Autodesk Fusion 360 part; units mm, degrees
(part 2 of 2)
sketch "Sketch53" plane through (0, 12.5, 0) normal (0, 1, 0) x (-1, 0, 0)
  circle A0 centre (-41, 14.5) radius 4.5
  line L0 (-2.4975, 53.5) -> (-2.4975, 22.5658)
  arc A1 (-31.7708, 34.6912) -> (-2.4975, 22.5658) centre (0.0025, 70) ccw
  line L1 (-31.7708, 34.6912) -> (-12.962, 53.5)
  line L2 (-12.962, 53.5) -> (-2.4975, 53.5)
  line L3 (12.9669, 53.5) -> (31.7757, 34.6912)
  arc A2 (2.5025, 22.5658) -> (31.7757, 34.6912) centre (0.0025, 70) ccw
  line L4 (2.5025, 22.5658) -> (2.5025, 53.5)
  line L5 (2.5025, 53.5) -> (12.9669, 53.5)
  line L6 (16.5025, 82.9645) -> (35.3113, 101.7733)
  arc A3 (47.4366, 72.5) -> (35.3113, 101.7733) centre (0.0025, 70) ccw
  line L7 (47.4366, 72.5) -> (16.5025, 72.5)
  line L8 (16.5025, 72.5) -> (16.5025, 82.9645)
  line L9 (-2.4975, 117.4342) -> (-2.4975, 86.5)
  line L10 (-2.4975, 86.5) -> (-12.962, 86.5)
  line L11 (-12.962, 86.5) -> (-31.7708, 105.3088)
  arc A4 (-2.4975, 117.4342) -> (-31.7708, 105.3088) centre (0.0025, 70) ccw
  line L12 (2.5025, 86.5) -> (2.5025, 117.4342)
  arc A5 (31.7757, 105.3088) -> (2.5025, 117.4342) centre (0.0025, 70) ccw
  line L13 (31.7757, 105.3088) -> (12.9669, 86.5)
  line L14 (12.9669, 86.5) -> (2.5025, 86.5)
  arc A6 (35.3113, 38.2267) -> (47.4366, 67.5) centre (0.0025, 70) ccw
  line L15 (35.3113, 38.2267) -> (16.5025, 57.0355)
  line L16 (16.5025, 57.0355) -> (16.5025, 67.5)
  line L17 (16.5025, 67.5) -> (47.4366, 67.5)
  line L18 (-47.4317, 67.5) -> (-16.4975, 67.5)
  line L19 (-16.4975, 67.5) -> (-16.4975, 57.0355)
  line L20 (-16.4975, 57.0355) -> (-35.3063, 38.2267)
  arc A7 (-47.4317, 67.5) -> (-35.3063, 38.2267) centre (0.0025, 70) ccw
  arc A8 (-35.3063, 101.7733) -> (-47.4317, 72.5) centre (0.0025, 70) ccw
  line L21 (-35.3063, 101.7733) -> (-16.4975, 82.9645)
  line L22 (-16.4975, 82.9645) -> (-16.4975, 72.5)
  line L23 (-16.4975, 72.5) -> (-47.4317, 72.5)
  line L24 (-50, 90) -> (-50, 0)
  line L25 (-50, 0) -> (53, 0)
  line L26 (53, 0) -> (53, 90)
  line L27 (53, 90) -> (50, 90)
  arc A9 (50, 90) -> (20, 120) centre (20, 90) ccw
  line L28 (20, 120) -> (-20, 120)
  arc A10 (-20, 120) -> (-50, 90) centre (-20, 90) ccw
  line L29 (50, 90) -> (58, 90)
  line L30 (58, 90) -> (58, 0)
  line L31 (58, 0) -> (50, 0)
  line L32 (50, 0) -> (50, 90)
  constraint horizontal L29
  constraint vertical L30
  constraint horizontal L31
  constraint vertical L32
  constraint coincident L27.end A9.start
extrude "Extrude57" add sketch "Sketch53" along normal blind 3 contours L25 L26 L27 L29 L31 L32 | L26 L29 L30 L31 bodies 1
sketch "Sketch54" plane through (0, 12.5, 0) normal (0, -1, 0) x (1, 0, 0)
  line L0 (-53, 0) -> (-53, 90)
  line L1 (-53, 90) -> (-58, 90)
  line L2 (-58, 90) -> (-58, 0)
  line L3 (-58, 0) -> (-53, 0)
  line L4 (-57.5, 90) -> (-55.5, 90)
  line L5 (-55.5, 90) -> (-55.5, 0)
  line L6 (-55.5, 0) -> (-57.5, 0)
  line L7 (-57.5, 0) -> (-57.5, 90)
  dimension "d272" = 0.5
  constraint perpendicular L4 L5
  constraint parallel L4 L6
  constraint parallel L5 L7
  constraint coincident L1 L4.end
  constraint coincident L1 L4.start
  measures "d272" distance of L2 L7
extrude "Extrude58" cut 1 faces at (53.8333, 12.5, 30) along direction (0, 1, 0) blind 1 on bodies 1 bodies 1
extrude "Extrude59" cut 1 faces at (57.6667, 12.5, 60) along direction (0, 1, 0) blind 1 on bodies 1 bodies 1
extrude "Extrude60" cut 1 faces at (54.6667, -12.5, 30) along direction (0, -1, 0) blind 1 on bodies 1 bodies 1
extrude "Extrude61" cut 1 faces at (57.6667, -12.5, 30) along direction (0, -1, 0) blind 1 on bodies 1 bodies 1
sketch "Sketch55" plane through (-50, 0, 0) normal (-1, 0, 0) x (0, -1, 0)
  line L0 (-10.5, 90) -> (-10.5, 0)
  line L1 (-10.5, 0) -> (10.5, 0)
  line L2 (10.5, 0) -> (10.5, 90)
  line L3 (10.5, 90) -> (-10.5, 90)
  line L4 (7.5, 30) -> (-7.5, 30)
  arc A0 (-7.5, 35) -> (-7.5, 30) centre (-7.5, 32.5) ccw
  line L5 (-7.5, 35) -> (7.5, 35)
  arc A1 (7.5, 30) -> (7.5, 35) centre (7.5, 32.5) ccw
  line L6 (-10.5, 2) -> (10.5, 2)
  dimension "d281" = 2
  constraint coincident L0 L6.start
  constraint coincident L2 L6.end
  constraint perpendicular L2 L6
  measures "d281" distance of L1 L6
extrude "Extrude62" add sketch "Sketch55" along normal blind 2 contours L0 L1 L2 L6 bodies 1
extrude "Extrude63" add 1 faces at (-52, 3.5, 0.6667) along direction (-1, 0, 0) blind 1 on bodies 1 bodies 1
sketch "Sketch56" plane through (76.5769, 0, 0) normal (1, 0, 0) x (0, 1, 0)
  line L0 (-61.7702, 35) -> (-46.7702, 35)
  arc A0 (-46.7702, 30) -> (-46.7702, 35) centre (-46.7702, 32.5) ccw
  line L1 (-46.7702, 30) -> (-61.7702, 30)
  arc A1 (-61.7702, 35) -> (-61.7702, 30) centre (-61.7702, 32.5) ccw
  line L2 (-46.7702, 75) -> (-61.7702, 75)
  arc A2 (-61.7702, 80) -> (-61.7702, 75) centre (-61.7702, 77.5) ccw
  line L3 (-61.7702, 80) -> (-46.7702, 80)
  arc A3 (-46.7702, 75) -> (-46.7702, 80) centre (-46.7702, 77.5) ccw
  line L4 (-61.7702, 50) -> (-46.7702, 50)
  arc A4 (-46.7702, 45) -> (-46.7702, 50) centre (-46.7702, 47.5) ccw
  line L5 (-46.7702, 45) -> (-61.7702, 45)
  arc A5 (-61.7702, 50) -> (-61.7702, 45) centre (-61.7702, 47.5) ccw
  line L6 (-61.7702, 65) -> (-46.7702, 65)
  arc A6 (-46.7702, 60) -> (-46.7702, 65) centre (-46.7702, 62.5) ccw
  line L7 (-46.7702, 60) -> (-61.7702, 60)
  arc A7 (-61.7702, 65) -> (-61.7702, 60) centre (-61.7702, 62.5) ccw
  line L8 (-66.7673, 2) -> (-64.7673, 2)
  line L9 (-64.7673, 2) -> (-64.7673, 25)
  line L10 (-64.7673, 25) -> (-43.7673, 25)
  line L11 (-43.7673, 25) -> (-43.7673, 2)
  line L12 (-43.7673, 2) -> (-41.7673, 2)
  line L13 (-41.7673, 2) -> (-41.7673, 85)
  arc A8 (-41.7673, 85) -> (-46.7673, 90) centre (-46.7673, 85) ccw
  line L14 (-46.7673, 90) -> (-61.7673, 90)
  arc A9 (-61.7673, 90) -> (-66.7673, 85) centre (-61.7673, 85) ccw
  line L15 (-66.7673, 85) -> (-66.7673, 2)
  line L16 (25, 44) -> (39, 44)
  line L17 (39, 40) -> (25, 40)
  arc A10 (39, 40) -> (39, 44) centre (39, 42) ccw
  arc A11 (25, 44) -> (25, 40) centre (25, 42) ccw
  dimension "d286" = 2
  constraint horizontal L16
  constraint horizontal L17
  constraint tangent L16 A10
  constraint tangent L17 A10
  constraint tangent L16 A11
  constraint tangent L17 A11
  measures "d286" radius of A10
extrude "Extrude64" add sketch "Sketch56" along normal blind 16 contours L16 L17 A10 A11 bodies 6 makes body 9
sketch "Sketch57" plane through (0, 0, 44) normal (0, 0, 1) x (-1, 0, 0)
  line L0 (-76.5769, -25) -> (-92.5769, -25)
  line L1 (-92.5769, -25) -> (-92.5769, -39)
  line L2 (-92.5769, -39) -> (-76.5769, -39)
  line L3 (-150.3526, 0.0058) -> (-149.3802, 0.0057)
  line L4 (-150.6028, -43.5952) -> (-149.3695, -43.5952)
  line L5 (-76.5769, -39) -> (-76.5769, -25)
  line L6 (-77.5769, -19.7473) -> (-76.5769, -19.7473)
  line L7 (-76.5769, -19.7473) -> (-76.5769, -43.4857)
  line L8 (-76.5769, -43.4857) -> (-77.5769, -43.4857)
  line L9 (-77.5769, -43.4857) -> (-77.5769, -19.7473)
  constraint horizontal L6
  constraint vertical L7
  constraint horizontal L8
  constraint perpendicular L6 L9
extrude "Extrude65" cut sketch "Sketch57" against normal blind 5 contours L0 L2 L5 L7 L9 | L0 L6 L7 L9 | L2 L7 L8 L9 bodies 9
sketch "Sketch58" plane through (92.5769, 0, 0) normal (1, 0, 0) x (0, 1, 0)
  line L0 (39, 44) -> (25, 44)
  arc A0 (25, 44) -> (25, 40) centre (25, 42) ccw
  line L1 (25, 40) -> (39, 40)
  line L2 (41, 45) -> (23, 45)
  line L3 (23, 39) -> (41, 39)
  arc A1 (23, 45) -> (23, 39) centre (23, 42) ccw
  arc A2 (41, 39) -> (41, 45) centre (41, 42) ccw
  arc A3 (39, 40) -> (39, 44) centre (39, 42) ccw
  dimension "d292" = 1
  dimension "d293" = 1
  dimension "d294" = 3
  constraint horizontal L2
  constraint tangent L2 A2
  constraint tangent L3 A2
  measures "d292" distance of L0 L2
  measures "d293" distance of L1 L3
  measures "d294" radius of A1
extrude "Extrude66" add sketch "Sketch58" along normal blind 3 contours L0 A0 L1 A3 | L2 L3 A1 A2 bodies 6 9
extrude "Extrude67" add sketch "Sketch54" along normal blind 2 contours L1 L3 L4 L5 L6 L7 bodies 1
extrude "Extrude68" cut 1 faces at (-54.6667, 12.5, 30) along direction (0, 1, 0) blind 1 on bodies 1 bodies 1
extrude "Extrude69" cut 1 faces at (-57.6667, 12.5, 30) along direction (0, 1, 0) blind 1 on bodies 1 bodies 1
extrude "Extrude70" cut 1 faces at (-54.6667, -12.5, 30) along direction (0, -1, 0) blind 1 on bodies 1 bodies 1
extrude "Extrude71" cut 1 faces at (-57.6667, -12.5, 30) along direction (0, -1, 0) blind 1 on bodies 1 bodies 1
move_body "Move12" bodies 9 to x (0, 0, -1) y (0, 1, 0) z (1, 0, 0) at (41.0769, 0, 96.0769)
copy_body "CopyPasteBodies4" bodies 9 makes body 10
move_body "Move13" bodies 10 to x (1, 0, 0) y (0, 1, 0) z (0, 0, 1) at (-13.0479, -30.5557, 0)
move_body "Move14" bodies 9 to x (1, 0, 0) y (0, 1, 0) z (0, 0, 1) at (-2.3285, -29.5516, 0)
move_body "Move15" bodies 8 7 6 to x (0, 0, 1) y (0, 1, 0) z (-1, 0, 0) at (146.8269, 0, -71.8269)
move_body "Move16" bodies 3 5 4 to x (0, 0, 1) y (0, -1, 0) z (1, 0, 0) at (61.4452, -217.8699, -50.3689)
move_body "Move19" bodies 8 to x (1, 0, 0) y (0, 1, 0) z (0, 0, 1) at (0.0422, -0.2059, 0)
move_body "Move17" bodies 10 9 to x (0, -1, 0) y (1, 0, 0) z (0, 0, 1) at (91.7101, -7.8168, 0)
move_body "Move18" bodies 1 to x (0, 0, 1) y (0, 1, 0) z (-1, 0, 0) at (84.3676, 0, 57.66)
